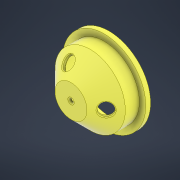
# Autodesk Inventor part: 016
Saved by Autodesk Inventor 2022 (Build 260153000, 153)
## iProperties
Created: 2021-11-15
Part Number: 016
Material: Stainless Steel, Austenitic
Document SubType Name: Modeling
Designer: vinicius.miguel
Density: 8 g/cm^3
Appearance: Smooth - Yellow
Author: vinicius.miguel
Autodesk Inventor part; units mm, degrees
ref_plane "YZ Plane" through (0, 0, 0) normal (1, 0, 0) x (0, 1, 0)
ref_plane "XZ Plane" through (0, 0, 0) normal (0, 1, 0) x (-1, 0, 0)
ref_plane "XY Plane" through (0, 0, 0) normal (0, 0, 1) x (1, 0, 0)
sketch "Sketch1" plane through (0, 0, 0) normal (0, 1, 0) x (-1, 0, 0)
  line L0 (1, -0.4) -> (4.5858, -0.4)
  line L1 (5, 0.6) -> (1, 0.6)
  arc A0 (1, 0.6) -> (1, -0.4) centre (1, 0.1) ccw
  line L2 (4.5858, -0.4) -> (10, -5.8142)
  line L3 (5, 0.6) -> (11, -5.4)
  line L4 (11, -5.4) -> (11, -9.8)
  line L5 (11, -9.8) -> (13, -9.8)
  line L6 (13, -9.8) -> (13, -11.3)
  line L7 (13, -11.3) -> (10, -11.3)
  line L8 (10, -11.3) -> (10, -5.8142)
  line L9 (0, 0) -> (0, -4.2235)
  dimension "d1" = 2
  dimension "d2" = 0.5
  dimension "d3" = 26
  dimension "d4" = 0.1
  dimension "d5" = 20
  dimension "d6" = 1
  dimension "d7" = 135
  dimension "d8" = 1
  dimension "d9" = 10
  dimension "d10" = 11.3
  dimension "d11" = 1.5
  constraints: 20 end point, 5 perpendicular, 2 parallel, 2 point on circle, 2 tangent, 2 vertical, 1 centre point
  measures "d1" diameter of A0.centre L9
  measures "d2" radius of A0
  measures "d3" diameter of L6 L9
  measures "d4" vertical distance of L9.start A0.centre
  measures "d5" diameter of L8 L9
  measures "d6" distance between parallel lines of L4 L8
  measures "d7" angle of L2 L0
  measures "d8" distance between parallel lines of L3 L2
  measures "d9" diameter of L1.start L9
  measures "d10" distance from line of L7 L9.start
  measures "d11" distance between parallel lines of L7 L5
revolve "Revolution1" add sketch "Sketch1" angle 360 about axis through (0, 0, 0) along (0, 0, -1)
sketch "Sketch2" plane through (0, 0, 0.6) normal (0, 0, 1) x (1, 0, 0)
  circle A0 centre (0, 0) radius 5 projected
  point P0 (5, 0)
  constraints: 2 horizontal alignment, 1 other
ref_plane "Work Plane1" through (5, 0, 0.6) normal (0.7071068, 0, 0.7071068) x (0, 1, 0)
sketch "Sketch3" plane through (5, 0, 0.6) normal (0.7071068, 0, 0.7071068) x (0, 1, 0)
  ellipse E0 centre (0, -0.7071) end of major axis (-11, -0.7071) minor radius 7.7782 projected
  ellipse E1 centre (0, 3.5355) end of major axis (-5, 3.5355) minor radius 3.5355 projected
  line L0 (0, -8.4853) -> (0, 0)
  point P0 (0, 3.1113)
  point P1 (0, -4.2426)
  constraints: 3 vertical alignment, 2 end point, 1 midpoint, 1 vertical, 2 other
hole "Hole1" at (8, 0, -2.4) direction (-0.7071068, 0, -0.7071068) diameter 4 end through all
fillet "Fillet1" radius 0.25 4 edges at (7.8321, 1.9991, -2.4832) (8.8676, -1.5054, -3.3945) (6.9891, -1.5059, -1.5495) (7.0614, 1.9957, -3.1522)
pattern_circular "Circular Pattern1" count 3 over 360 about axis through (0, 0, -7.6) along (0, 0, -1) of "Hole1", "Fillet1"
body "Solid1"
